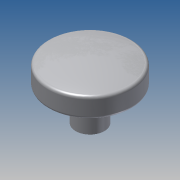
# Autodesk Inventor part: chimney
Saved by Autodesk Inventor 2014 SP1 (Build 180222100, 222)
## iProperties
Created: 2014-05-23
Part Number: chimney
Material: Aluminum 6061
Document SubType Name: Modeling
Designer: Dave
Density: 2.71 g/cm^3
Appearance: Aluminum - Flat
Mass: 2074.78 g
Surface Area: 9444.16 cm^2
Volume: 765.602 cm^3
Author: Dave
Autodesk Inventor part; units mm, degrees
ref_plane "YZ Plane" through (0, 0, 0) normal (1, 0, 0) x (0, 1, 0)
ref_plane "XZ Plane" through (0, 0, 0) normal (0, 1, 0) x (-1, 0, 0)
ref_plane "XY Plane" through (0, 0, 0) normal (0, 0, 1) x (1, 0, 0)
sketch "Sketch1" plane through (0, 0, 0) normal (0, 1, 0) x (-1, 0, 0)
  circle A0 centre (0, 0) radius 76.2
  circle A1 centre (0, 0) radius 74.93
  dimension "d0" = 152.4
  dimension "d1" = 1.27
  constraints: 2 centre point, 1 coincident
  measures "d0" diameter of A0
  measures "d1" radial gap between concentric circles of A1 A0
extrude "Extrusion1" add sketch "Sketch1" along normal blind 203.2
sketch "Sketch2" plane through (0, 203.2, 0) normal (0, 1, 0) x (1, 0, 0)
  circle A0 centre (0, 0) radius 74.93 projected
  circle A1 centre (0, 0) radius 76.2 projected
  point P0 (0, 76.2)
  constraints: 1 vertical alignment, 1 other
ref_plane "Work Plane1" through (0, 203.2, -76.2) normal (0, 0, -1) x (-1, 0, 0)
sketch "Sketch3" plane through (0, 203.2, -76.2) normal (0, 0, -1) x (-1, 0, 0)
  line L0 (-6.3336, -31.75) -> (6.3664, -31.75)
  line L1 (6.3664, -31.75) -> (6.3664, -12.7)
  line L2 (6.3664, -12.7) -> (-6.3336, -12.7)
  line L3 (-6.3336, -12.7) -> (-6.3336, -31.75)
  line L4 (76.2, 0) -> (-76.2, 0) projected
  point P0 (0, -203.2)
  point P1 (0.0164, -12.7)
  dimension "d4" = 12.7
  dimension "d5" = 19.05
  dimension "d6" = 12.7
  constraints: 8 end point, 2 parallel, 1 horizontal, 1 midpoint, 1 perpendicular
  measures "d4" distance of L0.start L0.end
  measures "d5" distance of L2.end L0.start
  measures "d6" distance between parallel lines of L2 L4
extrude "Extrusion2" add sketch "Sketch3" along normal blind 1.27
sketch "Sketch4" plane through (0, 203.2, -77.47) normal (0, 0, -1) x (-1, 0, 0)
  line L0 (-6.3336, -31.75) -> (6.3664, -31.75) projected
  line L1 (6.3664, -31.75) -> (6.3664, -12.7) projected
  line L2 (-6.3336, -31.75) -> (6.3664, -31.75)
  line L3 (6.3664, -31.75) -> (6.3664, -30.48)
  line L4 (6.3664, -30.48) -> (-6.3336, -30.48)
  line L5 (-6.3336, -30.48) -> (-6.3336, -31.75)
  point P0 (0, -203.2)
  dimension "d9" = 1.27
  constraints: 8 end point, 2 parallel, 1 horizontal, 1 perpendicular, 1 point on line
  measures "d9" distance between parallel lines of L2 L4
extrude "Extrusion3" add sketch "Sketch4" along normal blind 101.6
pattern_circular "Circular Pattern1" count 3 over 360 about axis through (0, -10, 0) along (0, 1, 0) of "Extrusion2", "Extrusion3"
ref_plane "Work Plane5" through (-0.0164, 171.45, -76.2) normal (1, 0, 0) x (0, 0, -1)
sketch "Sketch8" plane through (-0.0164, 171.45, -76.2) normal (1, 0, 0) x (0, 0, -1)
  arc A0 (143.3172, 90.1624) -> (129.3472, 104.1324) centre (129.3472, 90.1624) ccw
  line L0 (143.3172, 90.1624) -> (143.3172, 13.9624)
  arc A1 (129.3472, -0.0076) -> (143.3172, 13.9624) centre (129.3472, 13.9624) ccw
  line L1 (129.3472, -0.0076) -> (91.2472, -0.0076)
  line L2 (-76.2, 102.8624) -> (-76.2, -186.9408) construction
  line L3 (-76.2, 128.2624) -> (-2.5373, 128.2624) construction
  line L4 (-2.5373, 128.2624) -> (75.1026, 117.3507) construction
  line L5 (75.1026, 117.3507) -> (129.3472, 104.1324) construction
  spline S0 degree 3 poles (-76.2, 128.2624) (-2.5373, 128.2624) (75.1026, 117.3507) (129.3472, 104.1324) knots 1 1 1 1 2 2 2 2
  arc A2 (144.6472, 90.1624) -> (129.5104, 105.4616) centre (129.3472, 90.1624) ccw
  line L6 (144.6472, 90.1624) -> (144.6472, 13.9624)
  arc A3 (129.3472, -1.3376) -> (144.6472, 13.9624) centre (129.3472, 13.9624) ccw
  line L7 (129.3472, -1.3376) -> (91.2472, -1.3376)
  line L8 (91.2472, -1.3376) -> (91.2472, -0.0076)
  line L9 (-76.2, 129.5924) -> (-76.2, 128.2624)
  spline S1 degree 5 poles (-76.2, 129.5924) (-61.3628, 129.5924) (-46.5256, 129.2243) (-31.7005, 128.5331) (-2.6849, 126.5943) (26.2362, 123.56) (40.3703, 121.8221) (66.7891, 118.0958) (93.0572, 113.4287) (105.2649, 111.0344) (117.4252, 108.4029) (129.5104, 105.4616) knots 0 0 0 0 0 0 0.357413 0.357413 0.357413 0.700384 0.700384 0.700384 1 1 1 1 1 1
  point P0 (-76.2, -171.45)
  point P1 (142.0472, 1.2624)
  point P2 (142.0472, 102.8624)
  dimension "d27" = 101.6
  dimension "d39" = 25.4
  constraints: 14 end point, 8 point on circle, 4 centre point, 4 perpendicular, 1 concentric, 1 parallel, 9 other
  measures "d27" distance of point (142.047, 1.262) point (142.047, 102.862)
  measures "d39" distance of L2.start L3.start
revolve "Revolution3" add sketch "Sketch8" angle 360 about axis through (-0.0164, 274.3124, 0) along (0, -1, 0)
sketch "Sketch10" plane through (0, 203.2, 0) normal (0, 1, 0) x (1, 0, 0)
  circle A0 centre (0, 0) radius 82.55
  dimension "d34" = 165.1
  constraints: 1 centre point
  measures "d34" diameter of A0
extrude "Extrusion5" add sketch "Sketch10" along normal blind 6.35
sketch "Sketch11" plane through (0, 203.2, 0) normal (0, -1, 0) x (1, 0, 0)
  circle A0 centre (0, 0) radius 82.55 projected
  circle A1 centre (0, 0) radius 76.2 projected
extrude "Extrusion6" add sketch "Sketch11" along normal blind 12.7
body "Solid1"
